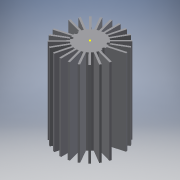
# Autodesk Inventor part: base
Saved by Autodesk Inventor 2018 (Build 220112000, 112)
## iProperties
Created: 2018-06-28
Part Number: base
Material: Generic
Document SubType Name: Modeling
Designer: David
Density: 1 g/cm^3
Appearance: Default
Author: David
Autodesk Inventor part; units mm, degrees
ref_plane "YZ Plane" through (0, 0, 0) normal (1, 0, 0) x (0, 1, 0)
ref_plane "XZ Plane" through (0, 0, 0) normal (0, 1, 0) x (-1, 0, 0)
ref_plane "XY Plane" through (0, 0, 0) normal (0, 0, 1) x (1, 0, 0)
sketch "Sketch1" plane through (0, 0, 0) normal (0, 0, 1) x (1, 0, 0)
  circle A0 centre (0, 0) radius 9.955
  dimension "d0" = 19.91
  constraints: 1 centre point, 1 coincident
  measures "d0" diameter of A0
extrude "Extrusion1" add sketch "Sketch1" along normal blind 40 and the other way blind 20
sketch "Sketch2" plane through (0, 0, 40) normal (0, 0, 1) x (1, 0, 0)
  circle A0 centre (0, 0) radius 9.955 projected
  circle A1 centre (9.955, 0) radius 1.215
  circle A2 centre (-9.955, 0) radius 1.215
  dimension "d3" = 2.43
  dimension "d4" = 2.43
  constraints: 2 centre point, 2 point on circle
  measures "d3" diameter of A1
  measures "d4" diameter of A2
extrude "Extrusion2" cut sketch "Sketch2" against normal blind 60 contours A0 A1 | A0 A1 | A2 A0 | A0 A2
sketch "Sketch3" plane through (0, 0, 40) normal (0, 0, 1) x (1, 0, 0)
  circle A0 centre (0, 0) radius 21.0058 construction
  line L0 (20.212, 5.72) -> (20.212, -5.72)
  line L1 (-20.212, 5.72) -> (-20.212, -5.72)
  line L2 (0, 0) -> (-20.212, 5.72) construction
  line L3 (-20.212, 5.72) -> (-20.3793, 5.0919)
  line L4 (-20.3793, 5.0919) -> (-9.7354, 2.0797)
  circle A1 centre (0, 0) radius 9.955 projected
  line L5 (-20.212, 5.72) -> (-20.0254, 6.3426)
  line L6 (-20.0254, 6.3426) -> (-9.3814, 3.3304)
  line L7 (-9.7354, 2.0797) -> (-9.3814, 3.3304)
  line L8 (0, 0) -> (-21.0058, 0) construction
  line L9 (-18.3954, 10.1416) -> (-8.878, 4.5037)
  line L10 (-8.878, 4.5037) -> (-8.2155, 5.6221)
  line L11 (-17.7329, 11.26) -> (-8.2155, 5.6221)
  line L12 (-18.0728, 10.7059) -> (-17.7329, 11.26)
  line L13 (-18.0728, 10.7059) -> (-18.3954, 10.1416)
  line L14 (-15.1844, 14.5148) -> (-7.4284, 6.6273)
  line L15 (-7.4284, 6.6273) -> (-6.5015, 7.5387)
  line L16 (-14.2575, 15.4262) -> (-6.5015, 7.5387)
  line L17 (-14.728, 14.9776) -> (-14.2575, 15.4262)
  line L18 (-14.728, 14.9776) -> (-15.1844, 14.5148)
  line L19 (-10.9603, 17.9197) -> (-5.4832, 8.3088)
  line L20 (-5.4832, 8.3088) -> (-4.3539, 8.9524)
  line L21 (-9.831, 18.5633) -> (-4.3539, 8.9524)
  line L22 (-10.4007, 18.2502) -> (-9.831, 18.5633)
  line L23 (-10.4007, 18.2502) -> (-10.9603, 17.9197)
  line L24 (-6.0052, 20.1291) -> (-3.1722, 9.436)
  line L25 (-3.1722, 9.436) -> (-1.9157, 9.7689)
  line L26 (-4.7487, 20.462) -> (-1.9157, 9.7689)
  line L27 (-5.3795, 20.3053) -> (-4.7487, 20.462)
  line L28 (-5.3795, 20.3053) -> (-6.0052, 20.1291)
  line L29 (-0.6494, 20.9958) -> (-0.6497, 9.9338)
  line L30 (-0.6497, 9.9338) -> (0.6502, 9.9337)
  line L31 (0.6505, 20.9957) -> (0.6502, 9.9337)
  line L32 (0.0006, 21.0058) -> (0.6505, 20.9957)
  line L33 (0.0006, 21.0058) -> (-0.6494, 20.9958)
  line L34 (4.7497, 20.4618) -> (1.9163, 9.7688)
  line L35 (1.9163, 9.7688) -> (3.1727, 9.4359)
  line L36 (6.0062, 20.1288) -> (3.1727, 9.4359)
  line L37 (5.3806, 20.305) -> (6.0062, 20.1288)
  line L38 (5.3806, 20.305) -> (4.7497, 20.4618)
  line L39 (9.832, 18.5627) -> (4.3543, 8.9522)
  line L40 (4.3543, 8.9522) -> (5.4836, 8.3085)
  line L41 (10.9613, 17.9191) -> (5.4836, 8.3085)
  line L42 (10.4016, 18.2497) -> (10.9613, 17.9191)
  line L43 (10.4016, 18.2497) -> (9.832, 18.5627)
  line L44 (14.2583, 15.4254) -> (6.5019, 7.5384)
  line L45 (6.5019, 7.5384) -> (7.4287, 6.6269)
  line L46 (15.1851, 14.514) -> (7.4287, 6.6269)
  line L47 (14.7288, 14.9769) -> (15.1851, 14.514)
  line L48 (14.7288, 14.9769) -> (14.2583, 15.4254)
  line L49 (17.7335, 11.259) -> (8.2158, 5.6216)
  line L50 (8.2158, 5.6216) -> (8.8782, 4.5032)
  line L51 (18.3959, 10.1406) -> (8.8782, 4.5032)
  line L52 (18.0734, 10.705) -> (18.3959, 10.1406)
  line L53 (18.0734, 10.705) -> (17.7335, 11.259)
  line L54 (20.0257, 6.3416) -> (9.3816, 3.3299)
  line L55 (9.3816, 3.3299) -> (9.7355, 2.0791)
  line L56 (20.3796, 5.0908) -> (9.7355, 2.0791)
  line L57 (20.2123, 5.7189) -> (20.3796, 5.0908)
  line L58 (20.2123, 5.7189) -> (20.0257, 6.3416)
  line L59 (-20.212, -5.72) -> (0, 0)
  line L60 (-20.212, -5.72) -> (-20.0254, -6.3426)
  line L61 (-20.212, -5.72) -> (-20.3793, -5.0919)
  line L62 (-20.3793, -5.0919) -> (-9.7354, -2.0797)
  circle A2 centre (0, 0) radius 9.955 projected
  line L63 (-20.0254, -6.3426) -> (-9.3814, -3.3304)
  line L64 (-9.7354, -2.0797) -> (-9.3814, -3.3304)
  line L65 (-18.3954, -10.1416) -> (-8.878, -4.5037)
  line L66 (-17.7329, -11.26) -> (-8.2155, -5.6221)
  circle A3 centre (0, 0) radius 21.0058 construction
  line L67 (-18.0728, -10.7059) -> (-17.7329, -11.26)
  line L68 (-18.0728, -10.7059) -> (-18.3954, -10.1416)
  line L69 (-8.878, -4.5037) -> (-8.2155, -5.6221)
  line L70 (-15.1844, -14.5148) -> (-7.4284, -6.6273)
  line L71 (-14.2575, -15.4262) -> (-6.5015, -7.5387)
  circle A4 centre (0, 0) radius 21.0058 construction
  line L72 (-14.728, -14.9776) -> (-14.2575, -15.4262)
  line L73 (-14.728, -14.9776) -> (-15.1844, -14.5148)
  line L74 (-7.4284, -6.6273) -> (-6.5015, -7.5387)
  line L75 (-10.9603, -17.9197) -> (-5.4832, -8.3088)
  line L76 (-9.831, -18.5633) -> (-4.3539, -8.9524)
  circle A5 centre (0, 0) radius 21.0058 construction
  line L77 (-10.4007, -18.2502) -> (-9.831, -18.5633)
  line L78 (-10.4007, -18.2502) -> (-10.9603, -17.9197)
  line L79 (-5.4832, -8.3088) -> (-4.3539, -8.9524)
  line L80 (-6.0052, -20.1291) -> (-3.1722, -9.436)
  line L81 (-4.7487, -20.462) -> (-1.9157, -9.7689)
  circle A6 centre (0, 0) radius 21.0058 construction
  line L82 (-5.3795, -20.3053) -> (-4.7487, -20.462)
  line L83 (-5.3795, -20.3053) -> (-6.0052, -20.1291)
  line L84 (-3.1722, -9.436) -> (-1.9157, -9.7689)
  line L85 (-0.6494, -20.9958) -> (-0.6497, -9.9338)
  line L86 (0.6505, -20.9957) -> (0.6502, -9.9337)
  circle A7 centre (0, 0) radius 21.0058 construction
  line L87 (0.0006, -21.0058) -> (0.6505, -20.9957)
  line L88 (0.0006, -21.0058) -> (-0.6494, -20.9958)
  line L89 (-0.6497, -9.9338) -> (0.6502, -9.9337)
  line L90 (4.7497, -20.4618) -> (1.9163, -9.7688)
  line L91 (6.0062, -20.1288) -> (3.1727, -9.4359)
  circle A8 centre (0, 0) radius 21.0058 construction
  line L92 (5.3806, -20.305) -> (6.0062, -20.1288)
  line L93 (5.3806, -20.305) -> (4.7497, -20.4618)
  line L94 (1.9163, -9.7688) -> (3.1727, -9.4359)
  line L95 (9.832, -18.5627) -> (4.3543, -8.9522)
  line L96 (10.9613, -17.9191) -> (5.4836, -8.3085)
  circle A9 centre (0, 0) radius 21.0058 construction
  line L97 (10.4016, -18.2497) -> (10.9613, -17.9191)
  line L98 (10.4016, -18.2497) -> (9.832, -18.5627)
  line L99 (4.3543, -8.9522) -> (5.4836, -8.3085)
  line L100 (14.2583, -15.4254) -> (6.5019, -7.5384)
  line L101 (15.1851, -14.514) -> (7.4287, -6.6269)
  circle A10 centre (0, 0) radius 21.0058 construction
  line L102 (14.7288, -14.9769) -> (15.1851, -14.514)
  line L103 (14.7288, -14.9769) -> (14.2583, -15.4254)
  line L104 (6.5019, -7.5384) -> (7.4287, -6.6269)
  line L105 (17.7335, -11.259) -> (8.2158, -5.6216)
  line L106 (18.3959, -10.1406) -> (8.8782, -4.5032)
  circle A11 centre (0, 0) radius 21.0058 construction
  line L107 (18.0734, -10.705) -> (18.3959, -10.1406)
  line L108 (18.0734, -10.705) -> (17.7335, -11.259)
  line L109 (8.2158, -5.6216) -> (8.8782, -4.5032)
  line L110 (20.0257, -6.3416) -> (9.3816, -3.3299)
  line L111 (20.3796, -5.0908) -> (9.7355, -2.0791)
  circle A12 centre (0, 0) radius 21.0058 construction
  line L112 (20.2123, -5.7189) -> (20.3796, -5.0908)
  line L113 (20.2123, -5.7189) -> (20.0257, -6.3416)
  line L114 (9.3816, -3.3299) -> (9.7355, -2.0791)
  point P0 (-9.8809, 1.2127)
  point P1 (9.8809, 1.2127)
  point P2 (9.8809, -1.2127)
  point P3 (-9.8809, -1.2127)
  point P4 (18.0728, 10.7059)
  point P5 (21.0028, -0.3525)
  point P6 (-21.0028, 0.3525)
  point P7 (-21.0037, -0.2975)
  point P8 (-20.9819, 1.0022)
  point P9 (-20.3051, -5.38)
  point P10 (14.728, 14.9776)
  point P11 (20.3926, 5.0385)
  point P12 (-20.3926, -5.0385)
  point P13 (-20.2269, -5.6671)
  point P14 (-20.5387, -4.4052)
  point P15 (-18.2499, -10.4011)
  point P16 (10.4007, 18.2502)
  point P17 (18.4219, 10.0934)
  point P18 (-18.4219, -10.0934)
  point P19 (-18.1008, -10.6586)
  point P20 (-18.7254, -9.5186)
  point P21 (-14.9773, -14.7284)
  point P22 (5.3795, 20.3053)
  point P23 (15.2223, 14.475)
  point P24 (-15.2223, -14.475)
  point P25 (-14.7672, -14.939)
  point P26 (-15.6629, -13.9971)
  point P27 (-10.7054, -18.0731)
  point P28 (-0.0006, 21.0058)
  point P29 (11.0072, 17.8909)
  point P30 (-11.0072, -17.8909)
  point P31 (-10.4484, -18.2229)
  point P32 (-11.5555, -17.5418)
  point P33 (-5.7195, -20.2122)
  point P34 (-5.3806, 20.305)
  point P35 (6.0578, 20.1133)
  point P36 (-6.0578, -20.1133)
  point P37 (-5.4326, -20.2911)
  point P38 (-6.6772, -19.9163)
  point P39 (-0.3519, -21.0029)
  point P40 (-10.4016, 18.2497)
  point P41 (0.7043, 20.994)
  point P42 (-0.7043, -20.994)
  point P43 (-0.0544, -21.0057)
  point P44 (-1.3536, -20.9621)
  point P45 (5.0391, -20.3924)
  point P46 (-14.7288, 14.9769)
  point P47 (-4.6962, 20.4741)
  point P48 (4.6962, -20.4741)
  point P49 (5.3274, -20.319)
  point P50 (4.0604, -20.6096)
  point P51 (10.0939, -18.4216)
  point P52 (-18.0734, 10.705)
  point P53 (-9.7834, 18.5884)
  point P54 (9.7834, -18.5884)
  point P55 (10.3538, -18.2768)
  point P56 (9.2035, -18.8822)
  point P57 (14.4754, -15.2219)
  point P58 (-20.2123, 5.7189)
  point P59 (-14.2179, 15.4627)
  point P60 (14.2179, -15.4627)
  point P61 (14.6895, -15.0154)
  point P62 (13.7327, -15.8952)
  point P63 (17.8912, -11.0067)
  dimension "d7" = 42.0116
  dimension "d8" = 11.44
  dimension "d9" = 11.44
  dimension "d10" = 0.65
  dimension "d11" = 0.65
  dimension "d16" = 148.4
  dimension "d18" = 0.65
  dimension "d19" = 0.65
  dimension "d22" = 148.4
  constraints: 230 end point, 4 point on circle, 3 parallel, 2 vertical, 1 coincident, 1 horizontal, 1 perpendicular, 403 other
  measures "d8" distance of L0.start L0.end
  measures "d9" distance of L1.start L1.end
  measures "d10" distance of L1.start L3.end
  measures "d11" distance of L1.start L5.end
  measures "d18" distance of L1.end L60.end
  measures "d19" distance of L1.end L61.end
extrude "Extrusion3" add sketch "Sketch3" against normal blind 60 contours L57 L56 L0 | L0 L56 A1 L54 L58 | L111 L112 L0 | L0 L113 L110 A1 L111 | L55 A1 | A1 L114 | L50 A1 | A1 L49 L53 L52 L51 | L106 L107 L108 L105 A1 | A1 L109 | L45 A1 | A1 L44 L48 L47 L46 | L101 L102 L103 L100 A1 | A1 L104 | L40 A1 | A1 L39 L43 L42 L41 | L96 L97 L98 L95 A1 | A1 L99 | L35 A1 | A1 L34 L38 L37 L36 | L91 L92 L93 L90 A1 | A1 L94 | L30 A1 | A1 L29 L33 L32 L31 | L86 L87 L88 L85 A1 | A1 L89 | L25 A1 | A1 L24 L28 L27 L26 | L81 L82 L83 L80 A1 | A1 L84 | L20 A1 | A1 L19 L23 L22 L21 | L76 L77 L78 L75 A1 | A1 L79 | L15 A1 | A1 L14 L18 L17 L16 | L71 L72 L73 L70 A1 | A1 L74 | L10 A1 | A1 L9 L13 L12 L11 | L66 L67 L68 L65 A1 | A1 L69 | A1 L4 L1 L5 L6 | L63 L60 L59 A1 | L4 L3 L1 | A1 L59 L1 L62 | L1 L61 L62
sketch "Sketch5" plane through (0, 0, 40) normal (0, 0, 1) x (1, 0, 0)
  point P0 (0, 0)
sketch "Sketch9" plane through (0, 0, 40) normal (0, 0, 1) x (1, 0, 0)
  point P0 (0, 0)
sketch "Sketch10" plane through (0, 0, 40) normal (0, 0, 1) x (1, 0, 0)
  circle A0 centre (8.23, 4.75) radius 1 projected
  circle A1 centre (-8.23, -4.75) radius 1 projected
  point P0 (0, 0)
extrude "Extrusion6" cut sketch "Sketch10" against normal blind 6
sketch "Sketch11" plane through (0, 0, -20) normal (0, 0, -1) x (-1, 0, 0)
  circle A0 centre (0, 0) radius 3
  dimension "d40" = 6
  constraints: 1 centre point, 1 coincident
  measures "d40" diameter of A0
extrude "Extrusion7" cut sketch "Sketch11" against normal blind 10
thread "Thread1" size "M6x1" class "6H" standard "ANSI Metric M Profile" full length
thread "Thread2" size "M2x0.4" class "6H" standard "ANSI Metric M Profile" full length
thread "Thread3" size "M2x0.4" class "6H" standard "ANSI Metric M Profile" full length
body "Solid1"
